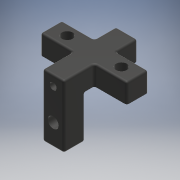
# Autodesk Inventor part: bed_spring_holder_back_v2
Saved by Autodesk Inventor 2018 (Build 220112000, 112)
## iProperties
Created: 2018-05-25
Part Number: bed_spring_holder_back_v2
Material: Plastic, Opaque Black
Document SubType Name: Modeling
Designer: Z. Deniz
Density: 0.952 g/cm^3
Appearance: Smooth - Black
Author: Z. Deniz
Autodesk Inventor part; units mm, degrees
ref_plane "YZ Plane" through (0, 0, 0) normal (1, 0, 0) x (0, 1, 0)
ref_plane "XZ Plane" through (0, 0, 0) normal (0, 1, 0) x (-1, 0, 0)
ref_plane "XY Plane" through (0, 0, 0) normal (0, 0, 1) x (1, 0, 0)
sketch "Sketch1" plane through (0, 0, 0) normal (1, 0, 0) x (0, 1, 0)
  line L0 (30, 0) -> (30, 9)
  line L1 (30, 9) -> (0, 9)
  line L2 (0, 9) -> (0, 0)
  line L3 (0, 0) -> (0, -20)
  line L4 (0, 0) -> (20, 0) construction
  line L5 (0, -20) -> (5, -20)
  line L6 (0, -20) -> (5, -20) construction
  line L7 (5, -20) -> (5, 0)
  line L8 (5, 0) -> (30, 0)
  line L9 (20, 9) -> (10, 9)
  line L10 (10, 9) -> (10, 0)
  line L11 (10, 0) -> (20, 0)
  line L12 (20, 0) -> (20, 9)
  line L13 (20, 9) -> (10, 0) construction
  line L14 (10, 9) -> (20, 0) construction
  point P0 (15, 4.5)
  dimension "d8" = 9
  dimension "d9" = 20
  dimension "d10" = 90
  dimension "d11" = 5
  dimension "d13" = 10
  dimension "d14" = 9
  dimension "d15" = 30
  dimension "d39" = 10
  constraints: 30 end point, 5 horizontal, 4 parallel, 3 perpendicular, 2 equal length, 2 midpoint, 2 point on line, 1 vertical
  measures "d8" distance of L0.end L0.start
  measures "d9" distance of L2.end L3.end
  measures "d10" angle of L3 L4
  measures "d11" distance of L3.end L5.end
  measures "d13" distance of L11.end L10.end
  measures "d14" distance of L11.end L9.start
  measures "d15" distance between parallel lines of L2 L0
  measures "d39" distance between parallel lines of L10 L2
extrude "Extrusion1" add sketch "Sketch1" along normal mid plane 10 contours L8 L12 L1 L0 | L8 L7 L5 L3 L2 L1 L10
extrude "Extrusion2" add sketch "Sketch1" along normal mid plane 40 contours L8 L10 L1 L12
fillet "Fillet1" radius 1 23 edges at (-5, 20, 4.5) (-5, 30, 4.5) (0, 30, 9) (-5, 2.5, -20) (5, 2.5, -20) (-5, 25, 9) (-12.5, 20, 9) (-20, 20, 4.5) (-20, 15, 9) (-20, 10, 4.5) (-12.5, 10, 9) (-5, 5, 9) (5, 5, 9) (12.5, 10, 9) (20, 15, 9) (20, 20, 4.5) (12.5, 20, 9) (5, 25, 9) (5, 20, 4.5) (5, 10, 4.5) (-5, 10, 4.5) (20, 10, 4.5) (5, 30, 4.5)
sketch "Sketch2" plane through (-4, 30, 8) normal (0, 1, 0) x (1, 0, 0)
  circle A0 centre (4, 3.5) radius 1.575
  line L0 (0, 8) -> (8, 8) projected
  line L1 (9, 8) -> (9, 0) projected
  line L2 (-1, 8) -> (-1, 0) projected
  point P0 (4, 8)
  dimension "d21" = 3.15
  dimension "d22" = 4.5
  dimension "d40" = 5
  constraints: 1 centre point
  measures "d21" diameter of A0
  measures "d22" distance from line of L0 A0.centre
  measures "d40" distance from line of L2 A0.centre
extrude "Extrusion3" cut sketch "Sketch2" against normal blind 35
sketch "Sketch3" plane through (-19, 19, 9) normal (0, 0, 1) x (1, 0, 0)
  circle A0 centre (6.5, -4) radius 2.5
  line L0 (-1, 0) -> (-1, -8) projected
  line L1 (13, 1) -> (0, 1) projected
  circle A1 centre (31.5, -4) radius 2.5
  line L2 (39, -8) -> (39, 0) projected
  line L3 (38, 1) -> (25, 1) projected
  point P0 (19, -19)
  dimension "d26" = 7.5
  dimension "d27" = 5
  dimension "d28" = 5
  dimension "d29" = 5
  dimension "d30" = 7.5
  dimension "d31" = 5
  constraints: 2 centre point
  measures "d26" distance from line of A0.centre L0
  measures "d27" distance from line of L1 A0.centre
  measures "d28" diameter of A1
  measures "d29" diameter of A0
  measures "d30" distance from line of L2 A1.centre
  measures "d31" distance from line of A1.centre L3
extrude "Extrusion4" cut sketch "Sketch3" against normal blind 9
sketch "Sketch4" plane through (-5, 5, 0) normal (0, 1, 0) x (1, 0, 0)
  circle A0 centre (5, 10) radius 2.5
  line L0 (1, 20) -> (9, 20) projected
  line L1 (0, 0) -> (0, 19) projected
  point P0 (5, 0)
  dimension "d34" = 5
  dimension "d35" = 10
  dimension "d36" = 5
  constraints: 1 centre point
  measures "d34" diameter of A0
  measures "d35" distance from line of L0 A0.centre
  measures "d36" distance from line of L1 A0.centre
extrude "Extrusion5" cut sketch "Sketch4" against normal blind 5
sketch "Sketch5" plane through (-4, 0, 9) normal (0, -1, 0) x (1, 0, 0)
  circle A0 centre (4, -19) radius 2.5 projected
  circle A1 centre (4, -4.5) radius 1.575 projected
  arc A2 (8, -29) -> (9, -28) centre (8, -28) ccw projected
  line L0 (9, -1) -> (9, -28) projected
  arc A3 (9, -1) -> (8, 0) centre (8, -1) ccw projected
  line L1 (0, 0) -> (8, 0) projected
  arc A4 (0, 0) -> (-1, -1) centre (0, -1) ccw projected
  line L2 (-1, -28) -> (-1, -1) projected
  arc A5 (-1, -28) -> (0, -29) centre (0, -28) ccw projected
  line L3 (0, -29) -> (8, -29) projected
  point P0 (4, -9)
extrude "Extrusion6" add sketch "Sketch5" along normal blind 4
fillet "Fillet2" radius 1 9 edges at (5, -4, -5.5) (4.7071, -4, 8.7071) (0, -4, 9) (-4.7071, -4, 8.7071) (-5, -4, -5.5) (-4.7071, -4, -19.7071) (0, -4, -20) (4.7071, -4, -19.7071) (0, 5, 0)
body "Solid1"
